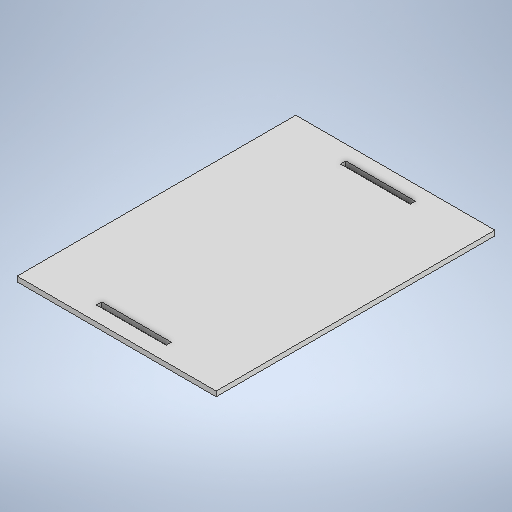
# Autodesk Inventor part: top
Saved by Autodesk Inventor 2025.3 (Build 293356030, 356C)
## iProperties
Created: 2026-06-26
Part Number: top
Material: Generic
Document SubType Name: Modeling
Designer: user
Density: 1 g/cm^3
Appearance: Default
Author: user
Autodesk Inventor part; units mm, degrees
ref_plane "YZ Plane" through (0, 0, 0) normal (1, 0, 0) x (0, 1, 0)
ref_plane "XZ Plane" through (0, 0, 0) normal (0, 1, 0) x (-1, 0, 0)
ref_plane "XY Plane" through (0, 0, 0) normal (0, 0, 1) x (1, 0, 0)
sketch "Sketch1" plane through (0, 0, 0) normal (0, 1, 0) x (-1, 0, 0)
  line L0 (0, 0) -> (-200, 0)
  line L1 (-200, 0) -> (-200, -280)
  line L2 (-200, -280) -> (0, -280)
  line L3 (0, -280) -> (0, 0)
  line L4 (-65, -14.7) -> (-135, -14.7)
  line L5 (-135, -14.7) -> (-135, -20)
  line L6 (-135, -20) -> (-65, -20)
  line L7 (-65, -20) -> (-65, -14.7)
  line L8 (-200, -140) -> (0, -140) construction
  line L9 (-65, -265.3) -> (-135, -265.3)
  line L10 (-135, -265.3) -> (-135, -260)
  line L11 (-135, -260) -> (-65, -260)
  line L12 (-65, -260) -> (-65, -265.3)
  line L13 (-200, -240) -> (-200, -40)
  dimension "d0" = 200
  dimension "d1" = 280
  dimension "d2" = 70
  dimension "d3" = 5.3
  constraints: 28 end point, 4 parallel, 4 symmetric about line, 2 horizontal, 2 midpoint, 2 perpendicular, 1 point on line
  measures "d0" distance of L2.end L1.end
  measures "d1" distance of L1.end L0.end
  measures "d2" distance of L6.end L5.end
  measures "d3" distance of L5.end L4.end
extrude "Extrusion1" add sketch "Sketch1" along normal blind 5
body "Solid1"
